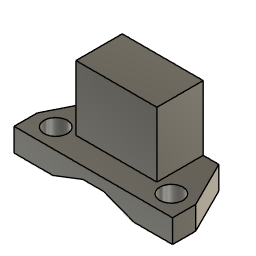
splayFlexJoint (Autodesk Fusion 360 archive; units mm, degrees)
design "hallEffectHolder"
Autodesk Fusion 360 part; units mm, degrees
note: some values were not read from the file. Chosen so that the rebuilt part matches the saved one: that a step has no effect; which face or edge a step refers to. Set by a fixed rule: which sketch regions a step uses.
sketch "mainBase" plane through (0, 0, 0) normal (0, 0, 1) x (1, 0, 0)
  line L0 (0, 0) -> (13.7, 0)
  line L1 (13.7, 0) -> (13.7, 6)
  line L2 (13.7, 6) -> (0, 6)
  line L3 (0, 6) -> (0, 0)
  line L4 (0, 0) -> (6.85, 0)
  line L5 (6.85, 0) -> (6.85, 1.75)
  line L6 (6.85, 1.75) -> (1.85, 1.75)
  line L7 (6.85, 1.75) -> (11.85, 1.75)
  line L8 (0, 6) -> (6.85, 6)
  circle A0 centre (1.85, 1.75) radius 1
  circle A1 centre (11.85, 1.75) radius 1
  line L9 (6.85, 6) -> (3.35, 6)
  line L10 (3.35, 6) -> (3.35, 2)
  line L11 (3.35, 2) -> (6.85, 2)
  line L12 (6.85, 2) -> (6.85, 6)
  line L13 (6.85, 6) -> (10.35, 6)
  line L14 (10.35, 6) -> (10.35, 2)
  line L15 (10.35, 2) -> (6.85, 2)
  line L16 (6.85, 2) -> (6.85, 6)
  dimension "d9" = 6
  dimension "d10" = 13.7
  dimension "d11" = 6.85
  dimension "d12" = 1.75
  dimension "d13" = 5
  dimension "d14" = 5
  dimension "d15" = 6.85
  dimension "d17" = 2
  dimension "d18" = 2
  dimension "d19" = 4
  dimension "d20" = 3.5
  dimension "d21" = 4
  dimension "d22" = 3.5
  constraint horizontal L0
  constraint vertical L1
  constraint horizontal L2
  constraint vertical L3
  constraint coincident L0.start L3.end
  constraint perpendicular L3 L4
  constraint perpendicular L0 L5
  constraint perpendicular L5 L6
  constraint perpendicular L5 L7
  constraint perpendicular L3 L8
  constraint coincident L6.end A0.centre
  constraint coincident L7.end A1.centre
  constraint horizontal L9
  constraint vertical L10
  constraint horizontal L11
  constraint vertical L12
  constraint horizontal L13
  constraint vertical L14
  constraint horizontal L15
  constraint vertical L16
  measures "d9" distance of L0.start L2.end
  measures "d10" distance of L0.start L0.end
  measures "d11" distance of L0.start L4.end
  measures "d12" distance of L4.end L5.end
  measures "d13" distance of L5.end L6.end
  measures "d14" distance of L5.end L7.end
  measures "d15" distance of L2.end L8.end
  measures "d17" diameter of A0
  measures "d18" diameter of A1
  measures "d19" distance of L8.end L11.end
  measures "d20" distance of L10.end L11.end
  measures "d21" distance of L8.end L11.end
  measures "d22" distance of L14.end L11.end
extrude "Extrude1" add sketch "mainBase" along normal blind 7.6 contours L2 L8 L9 L10 L11 L12 L16 | L2 L12 L13 L14 L15 L16
shell "Shell1" thickness 1 removed faces 1 at (8.0167, 4.6667, 0)
extrude "Extrude2" add sketch "mainBase" along normal blind 2 contours L0 L1 L2 L3 L4 L8 L10 L11 L14 L15
sketch "hallCutOut" plane through (0, 0, 0) normal (0, 0, 1) x (1, 0, 0)
  line L0 (0, 6) -> (6.85, 6)
  line L1 (6.85, 6) -> (6.85, 2)
  line L2 (6.85, 2) -> (3.35, 2)
  line L3 (3.35, 2) -> (3.35, 4)
  line L4 (6.85, 2) -> (6.85, 3)
  line L5 (6.85, 3) -> (5.95, 3)
  line L6 (5.95, 3) -> (3.35, 4)
  line L7 (6.85, 3) -> (7.75, 3)
  line L8 (6.85, 2) -> (10.35, 2)
  line L9 (10.35, 2) -> (10.35, 4)
  line L10 (10.35, 4) -> (7.75, 3)
  line L11 (7.75, 3) -> (9.35, 3)
  line L12 (9.35, 3) -> (9.35, 3.6154)
  line L13 (5.95, 3) -> (4.35, 3)
  line L14 (4.35, 3) -> (4.35, 3.6154)
  dimension "d31" = 6.85
  dimension "d32" = 4
  dimension "d33" = 3.5
  dimension "d34" = 2
  dimension "d35" = 1
  dimension "d36" = 0.9
  dimension "d37" = 0.9
  dimension "d38" = 3.5
  dimension "d39" = 2
  constraint horizontal L0
  constraint perpendicular L0 L1
  constraint perpendicular L1 L2
  constraint perpendicular L2 L3
  constraint perpendicular L2 L4
  constraint perpendicular L1 L5
  constraint perpendicular L1 L7
  constraint perpendicular L4 L8
  constraint perpendicular L8 L9
  constraint parallel L7 L11
  constraint coincident L10 L12.end
  constraint perpendicular L11 L12
  constraint perpendicular L1 L13
  constraint coincident L6 L14.end
  constraint perpendicular L13 L14
  measures "d31" distance of L0.start L0.end
  measures "d32" distance of L0.end L1.end
  measures "d33" distance of L1.end L2.end
  measures "d34" distance of L2.end L3.end
  measures "d35" distance of L1.end L4.end
  measures "d36" distance of L4.end L5.end
  measures "d37" distance of L4.end L7.end
  measures "d38" distance of L1.end L8.end
  measures "d39" distance of L8.end L9.end
extrude "Extrude3" add sketch "hallCutOut" along normal blind 6.6 contours L6 L13 L14 | L10 L11 L12
sketch "wireCutOut" plane through (0, 0, 0) normal (0, -1, 0) x (1, 0, 0)
  line L0 (0, 0) -> (13.7, 0)
  line L1 (13.7, 0) -> (13.7, 2)
  line L2 (13.7, 2) -> (0, 2)
  line L3 (0, 2) -> (0, 0)
  line L4 (0, 0) -> (6.85, 0)
  line L5 (6.85, 0) -> (6.85, 1)
  line L6 (6.85, 1) -> (5.95, 1)
  line L7 (6.85, 1) -> (7.75, 1)
  line L8 (6.85, 0) -> (13.7, 0)
  line L9 (6.85, 0) -> (10.35, 0)
  line L10 (6.85, 0) -> (3.35, 0)
  line L11 (7.75, 1) -> (10.35, 0)
  line L12 (5.95, 1) -> (3.35, 0)
  dimension "d42" = 6.85
  dimension "d43" = 1
  dimension "d44" = 0.9
  dimension "d45" = 0.9
  dimension "d46" = 6.85
  dimension "d47" = 3.5
  dimension "d48" = 3.5
  constraint coincident L0.start L3.end
  constraint perpendicular L3 L4
  constraint perpendicular L4 L5
  constraint perpendicular L5 L6
  constraint perpendicular L5 L7
  constraint perpendicular L5 L8
  constraint perpendicular L5 L9
  constraint perpendicular L5 L10
  measures "d42" distance of L0.start L4.end
  measures "d43" distance of L4.end L5.end
  measures "d44" distance of L5.end L6.end
  measures "d45" distance of L5.end L7.end
  measures "d46" distance of L4.end L0.end
  measures "d47" distance of L4.end L9.end
  measures "d48" distance of L4.end L10.end
extrude "Extrude4" cut sketch "wireCutOut" against normal blind 5 contours L0 L4 L5 L6 L10 L12 | L0 L5 L7 L8 L9 L11
sketch "cutOut" plane through (0, 0, 0) normal (0, 0, 1) x (1, 0, 0)
  line L0 (0, 0) -> (13.7, 0)
  line L1 (13.7, 0) -> (13.7, 6)
  line L2 (13.7, 6) -> (0, 6)
  line L3 (0, 6) -> (0, 0)
  line L4 (13.7, 0) -> (13.7, 2)
  line L5 (0, 0) -> (0, 2)
  line L6 (0, 6) -> (2, 6)
  line L7 (13.7, 6) -> (11.7, 6)
  line L8 (0, 2) -> (2, 6)
  line L9 (13.7, 2) -> (11.7, 6)
  dimension "d51" = 6
  dimension "d52" = 13.7
  dimension "d53" = 2
  dimension "d54" = 2
  dimension "d55" = 2
  dimension "d56" = 2
  constraint horizontal L0
  constraint vertical L1
  constraint horizontal L2
  constraint vertical L3
  constraint coincident L0.start L3.end
  constraint perpendicular L0 L4
  constraint perpendicular L0 L5
  constraint coincident L2 L6.end
  constraint perpendicular L1 L7
  measures "d51" distance of L0.start L2.end
  measures "d52" distance of L0.start L0.end
  measures "d53" distance of L0.end L4.end
  measures "d54" distance of L0.start L5.end
  measures "d55" distance of L1.end L7.end
  measures "d56" distance of L2.end L6.end
extrude "Extrude5" cut sketch "cutOut" along normal blind 2 contours L2 L3 L6 L8 | L1 L2 L7 L9
equation "baseLength = 6 mm"
equation "baseWidth = 13.7 mm"
equation "mountingCircleToMountingCircle = 10 mm"
equation "mountingHoleFromEdge = 1.75 mm"
equation "hallEffectWidth = 7 mm"
equation "hallEffectLength = 4 mm"
equation "hallEffectHeight = 7.6 mm"
equation "baseHeight = 2 mm"
equation "d9 = baseLength"
equation "d10 = baseWidth"
equation "d11 = baseWidth / 2"
equation "d12 = mountingHoleFromEdge"
equation "d13 = mountingCircleToMountingCircle / 2"
equation "d14 = mountingCircleToMountingCircle / 2"
equation "d15 = baseWidth / 2"
equation "screwHole = 2 mm"
equation "d17 = screwHole"
equation "d18 = screwHole"
equation "d19 = hallEffectLength"
equation "d20 = hallEffectWidth / 2"
equation "d21 = hallEffectLength"
equation "d22 = hallEffectWidth / 2"
equation "d23 = hallEffectHeight"
equation "hallEffectThickness = 1 mm"
equation "d26 = hallEffectThickness"
equation "d27 = baseHeight"
equation "traingleHeight = 2 mm"
equation "hallEffectMiddleDist = 1.8 mm"
equation "d31 = baseWidth / 2"
equation "d32 = hallEffectLength"
equation "d33 = hallEffectWidth / 2"
equation "d34 = traingleHeight"
equation "d35 = hallEffectThickness"
equation "d36 = hallEffectMiddleDist / 2"
equation "d37 = hallEffectMiddleDist / 2"
equation "d38 = hallEffectWidth / 2"
equation "d39 = traingleHeight"
equation "d40 = hallEffectHeight - hallEffectThickness"
equation "d42 = baseWidth / 2"
equation "d43 = hallEffectThickness"
equation "d44 = hallEffectMiddleDist / 2"
equation "d45 = hallEffectMiddleDist / 2"
equation "d46 = baseWidth / 2"
equation "d47 = hallEffectWidth / 2"
equation "d48 = hallEffectWidth / 2"
equation "d49 = -( baseLength - hallEffectThickness )"
equation "d51 = baseLength"
equation "d52 = baseWidth"
equation "d53 = baseLength / 3"
equation "d54 = baseLength / 3"
equation "d57 = baseHeight"

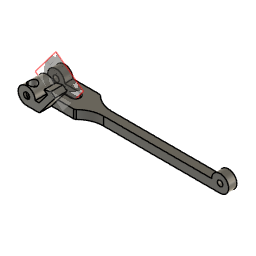
design "bar2Magnet"
Autodesk Fusion 360 part; units mm, degrees
sketch "mainBody" plane through (0, 0, 0) normal (0, 0, 1) x (1, 0, 0)
  line L0 (0, 0) -> (50, 0)
  line L1 (50, 0) -> (50, -1.5)
  line L2 (50, -1.5) -> (0, -1.5)
  line L3 (0, -1.5) -> (0, 0)
  line L4 (0, 0) -> (50, 0)
  line L5 (50, 0) -> (50, 1.5)
  line L6 (50, 1.5) -> (0, 1.5)
  line L7 (0, 1.5) -> (0, 0)
  line L8 (0, 0) -> (-4.4, 0)
  line L9 (-4.4, 0) -> (-4.4, 4.7)
  line L10 (-4.4, 4.7) -> (0, 4.7)
  line L11 (0, 4.7) -> (0, 0)
  line L12 (0, 0) -> (-4.4, 0)
  line L13 (-4.4, 0) -> (-4.4, -4.7)
  line L14 (-4.4, -4.7) -> (0, -4.7)
  line L15 (0, -4.7) -> (0, 0)
  line L16 (-4.4, -4.7) -> (-13.2, -4.7)
  line L17 (-13.2, -4.7) -> (-13.2, -1.7)
  line L18 (-13.2, -1.7) -> (-4.4, -1.7)
  line L19 (-4.4, -1.7) -> (-4.4, -4.7)
  line L20 (-4.4, 4.7) -> (-13.2, 4.7)
  line L21 (-13.2, 4.7) -> (-13.2, 1.7)
  line L22 (-13.2, 1.7) -> (-4.4, 1.7)
  line L23 (-4.4, 1.7) -> (-4.4, 4.7)
  line L24 (50, -1.5) -> (46.25, -1.5)
  line L25 (46.25, -1.5) -> (39.25, -1.5)
  line L26 (39.25, -1.5) -> (39.25, -0.5)
  line L27 (39.25, -0.5) -> (46.25, -0.5)
  line L28 (46.25, -0.5) -> (46.25, -1.5)
  dimension "d10" = 1.5
  dimension "d11" = 50
  dimension "d12" = 50
  dimension "d13" = 1.5
  dimension "d14" = 4.7
  dimension "d15" = 4.7
  dimension "d16" = 4.4
  dimension "d17" = 4.4
  dimension "d18" = 3
  dimension "d19" = 8.8
  dimension "d20" = 8.8
  dimension "d21" = 3
  dimension "d25" = 3.75
  dimension "d26" = 1
  dimension "d27" = 7
  dimension "d68" = 3.4
  constraint horizontal L0
  constraint vertical L1
  constraint horizontal L2
  constraint vertical L3
  constraint coincident L0.start L3.end
  constraint horizontal L4
  constraint vertical L5
  constraint horizontal L6
  constraint vertical L7
  constraint horizontal L8
  constraint vertical L9
  constraint horizontal L10
  constraint vertical L11
  constraint horizontal L12
  constraint vertical L13
  constraint horizontal L14
  constraint vertical L15
  constraint horizontal L16
  constraint vertical L17
  constraint horizontal L18
  constraint vertical L19
  constraint horizontal L20
  constraint vertical L21
  constraint horizontal L22
  constraint vertical L23
  constraint perpendicular L1 L24
  constraint horizontal L25
  constraint vertical L26
  constraint horizontal L27
  constraint vertical L28
  measures "d10" distance of L0.start L2.end
  measures "d11" distance of L1.end L2.end
  measures "d12" distance of L5.end L6.end
  measures "d13" distance of L0.start L6.end
  measures "d14" distance of L0.start L10.end
  measures "d15" distance of L0.start L14.end
  measures "d16" distance of L9.end L10.end
  measures "d17" distance of L13.end L14.end
  measures "d18" distance of L13.end L18.end
  measures "d19" distance of L13.end L16.end
  measures "d20" distance of L9.end L20.end
  measures "d21" distance of L20.end L21.end
  measures "d25" distance of L1.end L24.end
  measures "d26" distance of L24.end L27.end
  measures "d27" distance of L24.end L25.end
  measures "d68" distance of L18.end L22.end
extrude "Extrude1" add sketch "mainBody" along normal blind 3.125 contours L0 L4 L5 L6 L7 L11 | L0 L1 L2 L3 L4 L15 L24 L26 L27 L28 | L7 L8 L9 L10 L11 L12 L23 | L3 L8 L12 L13 L14 L15 L19 | L9 L20 L21 L22 L23 | L13 L16 L17 L18 L19
sketch "backHole" plane through (0, -1.5, 0) normal (0, -1, 0) x (1, 0, 0)
  line L0 (0, 0) -> (39.25, 0)
  line L1 (39.25, 0) -> (39.25, 3.125)
  line L2 (39.25, 3.125) -> (0, 3.125)
  line L3 (0, 3.125) -> (0, 0)
  circle A0 centre (50, 3.125) radius 3.125
  circle A1 centre (50, 3.125) radius 1
  line L4 (0, 0) -> (50, 0)
  line L5 (50, 0) -> (50, 3.125)
  line L6 (50, 3.125) -> (0, 3.125)
  line L7 (0, 3.125) -> (0, 0)
  dimension "d30" = 6.25
  dimension "d31" = 2
  dimension "d65" = 50
  dimension "d66" = 3.125
  constraint concentric A0 A1
  constraint horizontal L4
  constraint vertical L5
  constraint horizontal L6
  constraint vertical L7
  constraint coincident A0.centre A1.centre
  constraint coincident L0.start L3.end
  measures "d30" diameter of A0
  measures "d31" diameter of A1
  measures "d65" distance of L0.start L4.end
  measures "d66" distance of L0.start L2.end
extrude "Extrude2" cut sketch "backHole" against normal blind 3 contours A1 L5 L6 | A1 L5 L6
extrude "Extrude3" add sketch "backHole" against normal blind 3 contours A0 A1 L5 L6 | A0 A1 L5 L6
sketch "oneFrontHole" plane through (0, -1.7, 0) normal (0, 1, 0) x (-1, 0, 0)
  line L0 (4.4, 0) -> (13.2, 0)
  line L1 (13.2, 0) -> (13.2, 3.125)
  line L2 (13.2, 3.125) -> (4.4, 3.125)
  line L3 (4.4, 3.125) -> (4.4, 0)
  circle A0 centre (13.2, 3.125) radius 3.125
  circle A1 centre (13.2, 3.125) radius 1.1
  line L4 (13.2, 0) -> (0, 0)
  dimension "d40" = 6.25
  dimension "d41" = 2.2
  dimension "d74" = 13.2
  dimension "d75" = 3.125
  constraint coincident L1.end L2.start
  constraint concentric A0 A1
  measures "d40" diameter of A0
  measures "d41" diameter of A1
  measures "d74" distance of L0.end L4.end
  measures "d75" distance of L0.end L1.end
extrude "Extrude4" cut sketch "oneFrontHole" against normal blind 3 contours L1 L2 A1 picked at (12.4704, 3.0728)
extrude "Extrude5" add sketch "oneFrontHole" against normal blind 3 contours L1 L2 A0 A1 picked at (12.4537, 5.4515)
sketch "twoFrontHole" plane through (0, 1.7, 0) normal (0, -1, 0) x (1, 0, 0)
  line L0 (-13.2, 0) -> (-4.4, 0)
  line L1 (-4.4, 0) -> (-4.4, 3.125)
  line L2 (-4.4, 3.125) -> (-13.2, 3.125)
  line L3 (-13.2, 3.125) -> (-13.2, 0)
  circle A0 centre (-13.2, 3.125) radius 3.125
  circle A1 centre (-13.2, 3.125) radius 1.1
  dimension "d46" = 6.25
  dimension "d47" = 2.2
  constraint coincident L2.end L3.start
  measures "d46" diameter of A0
  measures "d47" diameter of A1
extrude "Extrude6" cut sketch "twoFrontHole" against normal blind 3 contours L2 L3 A1 picked at (-12.4704, 3.0728)
extrude "Extrude7" add sketch "twoFrontHole" against normal blind 3 contours L2 L3 A0 A1 picked at (-14.7245, 1.2154)
extrude "Extrude8" add sketch "mainBody" along normal blind 3.125 contours L2 L25 L26 L27 L28
fillet "Fillet1" radius 10 1 edges at (0, -1.5, 1.5625)
fillet "Fillet2" radius 10 1 edges at (0, 1.5, 1.5625)
fillet "Fillet3" radius 1 2 edges at (0, 4.7, 1.5625) (0, -4.7, 1.5625)
fillet "Fillet4" [no effect]
fillet "Fillet5" [no effect]
sketch "roundedInside" plane through (0, 0, 3.125) normal (0, 0, 1) x (-1, 0, 0)
  line L0 (10.075, -4.7) -> (10.075, -1.7)
  line L1 (10.075, -1.7) -> (4.4, -1.7)
  line L2 (4.4, -1.7) -> (4.4, 1.7)
  line L3 (4.4, 1.7) -> (10.075, 1.7)
  line L4 (10.075, 1.7) -> (10.075, 4.7)
  line L5 (-46.875, 1.5) -> (-46.875, -1.5)
  circle A0 centre (4.4, 0) radius 1.7
  arc A1 (0.4242, 4.7) -> (-0.281, 4.4091) centre (0.4242, 3.7) ccw
  arc A2 (-7.3321, 1.5) -> (-0.281, 4.4091) centre (-7.3321, 11.5) ccw
  line L6 (-7.3321, 1.5) -> (-46.875, 1.5)
  line L7 (-46.875, -1.5) -> (-7.3321, -1.5)
  arc A3 (-0.281, -4.4091) -> (-7.3321, -1.5) centre (-7.3321, -11.5) ccw
  arc A4 (-0.281, -4.4091) -> (0.4242, -4.7) centre (0.4242, -3.7) ccw
  line L8 (0.4242, -4.7) -> (10.075, -4.7)
  line L9 (10.075, 4.7) -> (0.4242, 4.7)
  dimension "d69" = 3.4
  constraint midpoint L2 A0.centre
  measures "d69" diameter of A0
extrude "Extrude9" cut sketch "roundedInside" against normal blind 3.125 contours L2 A0 | L2 A0
fillet "Fillet6" [no effect]
sketch "magnet" plane through (0, -4.7, 0) normal (0, -1, 0) x (1, 0, 0)
  line L0 (-0.4242, 0) -> (-0.4242, 3.125)
  line L1 (-0.4242, 3.125) -> (-10.075, 3.125)
  arc A0 (-10.075, 3.125) -> (-13.2, 0) centre (-13.2, 3.125) ccw
  line L2 (-13.2, 0) -> (-0.4242, 0)
  circle A1 centre (-13.2, 3.125) radius 1.1
  line L3 (0, 0) -> (-13.2, 0)
  line L4 (-13.2, 0) -> (-13.2, 3.125)
  line L5 (-13.2, 3.125) -> (0, 3.125)
  line L6 (0, 3.125) -> (0, 0)
  circle A2 centre (-13.2, 3.125) radius 3.125
  dimension "d76" = 6.25
  constraint horizontal L3
  constraint vertical L4
  constraint horizontal L5
  constraint vertical L6
  constraint coincident A0.centre A1.centre
  constraint coincident L3.start L6.end
  constraint concentric A0 A2
  measures "d76" diameter of A2
extrude "Extrude10" add sketch "magnet" along normal blind 4.4 contours A0 A1 L4 L5 A2 | A1 L4 L5 A2 | A1 L4 L5 | A1 L4 L5
hole "Hole1" at (-15.4097, -6.754, 5.3347) direction (0.707107, 0, -0.707107) diameter 1 depth 4 tip angle 180
extrude "Extrude11" add 1 faces at (-12.374, -9.1, 3.2495) along direction (0, 1, 0) blind 4.4
hole "Hole2" at (-10.9903, -6.7983, 5.3347) direction (-0.707107, 0, -0.707107) diameter 3.2 depth 7.8 tip angle 180
sketch "Sketch9" plane through (0, -4.7, 0) normal (0, -1, 0) x (1, 0, 0)
  arc A0 (-13.2, 0) -> (-10.075, 3.125) centre (-13.2, 3.125) ccw
  line L0 (-13.2, 0) -> (-0.4242, 0)
  line L1 (-0.4242, 0) -> (-0.4242, 3.125)
  line L2 (-0.4242, 3.125) -> (-10.075, 3.125)
  line L3 (-10.075, 3.125) -> (-13, 0)
  line L4 (-13, 0) -> (-11, 0)
  line L5 (-10.075, 3.125) -> (-8.075, 3.125)
  line L6 (-11, 0) -> (-8.075, 3.125)
  line L7 (-10.075, 3.125) -> (-4.4181, 8.7819)
  line L8 (-8.075, 3.125) -> (-2.6081, 8.9657)
  line L9 (-4.4181, 8.7819) -> (-2.6081, 8.9657)
  line L10 (-4.4181, 8.7819) -> (-5.8324, 10.1961)
  line L11 (-2.6081, 8.9657) -> (-5.8324, 10.1961)
  dimension "d92" = 2
  dimension "d93" = 2
  dimension "d95" = 8
  dimension "d96" = 8
  dimension "d98" = 2
  constraint coincident A0.end L2.end
  constraint coincident L0 L3.end
  constraint parallel L0 L4
  constraint parallel L2 L5
  constraint parallel L6 L8
  constraint perpendicular L7 L10
  measures "d92" distance of L3.end L4.end
  measures "d93" distance of A0.end L5.end
  measures "d95" distance of A0.end L7.end
  measures "d96" distance of L5.end L8.end
  measures "d98" distance of L7.end L10.end
extrude "Extrude12" add sketch "Sketch9" along normal blind 4.4 contours A0 L0 L2 L3 L4 L5 L6 | L2 L5 L7 L8 L9 | L9 L10 L11
extrude "Extrude13" add sketch "magnet" along normal blind 4.4 contours A0 A1 L4 L5 A2 | A1 L4 L5 A2 | A1 L4 L5 | A1 L4 L5
hole "Hole3" at (-13.2, -7.0048, 0) direction (0, 0, 1) diameter 3.2 depth 6.25 tip angle 180
extrude "Extrude14" cut 1 faces at (-13.5393, -4.7, 3.4906) along direction (0, -1, 0) blind 4.4
extrude "Extrude15" cut sketch "Sketch9" along normal blind 4.4 contours A0 L0 L2 L3 L4 L5 L6 | L2 L5 L7 L8 L9 | L9 L10 L11
sketch "Sketch12" plane through (0, -4.7, 0) normal (0, -1, 0) x (1, 0, 0)
  line L0 (-13.2, 0) -> (-0.4242, 0)
  line L1 (-0.4242, 0) -> (-0.4242, 3.125)
  line L2 (-0.4242, 3.125) -> (-10.075, 3.125)
  arc A0 (-13.2, 0) -> (-10.075, 3.125) centre (-13.2, 3.125) ccw
  line L3 (-5.675, 7.2) -> (-8.0564, 4.0395)
  line L4 (-8.0564, 4.0395) -> (-13.6194, 8.2311)
  line L5 (-13.6194, 8.2311) -> (-11.2359, 11.3943)
  line L6 (-11.2359, 11.3943) -> (-5.675, 7.2)
  line L7 (-5.675, 7.2) -> (-5.575, 7.2)
  line L8 (-5.575, 7.2) -> (-8, 4)
  line L9 (-8, 4) -> (-11.0312, 0)
  line L10 (-11.2359, 11.3943) -> (-11.2359, 11.4943)
  line L11 (-5.575, 7.2) -> (-4.3663, 8.7934)
  line L12 (-5.575, 7.2) -> (-3.9816, 5.9913)
  line L13 (-3.9816, 5.9913) -> (-2.7729, 7.5847)
  line L14 (-3.9816, 5.9913) -> (-8.5265, 0)
  line L15 (-8.5265, 0) -> (-11.0312, 0)
  line L16 (-5.575, 7.2) -> (-6.8689, 8.1816)
  line L17 (-6.8689, 8.1816) -> (-4.3663, 8.7934)
  line L18 (-4.3663, 8.7934) -> (-2.7729, 7.5847)
  dimension "d111" = 0.1
  dimension "d112" = 0.1
  dimension "d115" = 2
  dimension "d116" = 2
  dimension "d117" = 2
  constraint perpendicular L3 L4
  constraint perpendicular L4 L5
  constraint horizontal L7
  constraint coincident L0 L9.end
  constraint parallel L8 L9
  constraint vertical L10
  constraint perpendicular L11 L12
  constraint perpendicular L12 L13
  constraint coincident L0 L14.end
  constraint perpendicular L12 L14
  constraint perpendicular L11 L16
  measures "d111" distance of L3.start L7.end
  measures "d112" distance of L5.end L10.end
  measures "d115" distance of L7.end L11.end
  measures "d116" distance of L7.end L12.end
  measures "d117" distance of L12.end L13.end
extrude "Extrude16" add sketch "Sketch12" along normal blind 4.4 contours L0 L2 A0 L9 | L0 L2 L9 L14 L15 | L2 L8 L9 L12 L14 | L11 L12 L13 L18 | L11 L16 L17
hole "Hole4" at (-13.2, -7.0134, 6.25) direction (0, 0, -1) diameter 3.2 depth 7 tip angle 118
equation "mainBarLength = 50 mm" comment "50mm"
equation "mainBarWidth = 3 mm"
equation "mainBarHeight = 3.125 mm"
equation "tBarLength = 9.4 mm"
equation "tBarWidth = 4.4 mm"
equation "hBarHeight = 8.8 mm" comment "6.8mm"
equation "hBarWidth = 3 mm"
equation "outerCircle = 6.25 mm"
equation "innerCircle = 2.2 mm"
equation "d10 = mainBarWidth / 2"
equation "d11 = mainBarLength"
equation "d12 = mainBarLength"
equation "d13 = mainBarWidth / 2"
equation "d14 = tBarLength / 2"
equation "d15 = tBarLength / 2"
equation "d16 = tBarWidth"
equation "d17 = tBarWidth"
equation "d18 = hBarWidth"
equation "d19 = hBarHeight"
equation "d20 = hBarHeight"
equation "d21 = hBarWidth"
equation "insertDist = 3.75 mm"
equation "insertWidth = 7 mm"
equation "insertHeight = 1 mm"
equation "d25 = insertDist"
equation "d26 = insertHeight"
equation "d27 = insertWidth"
equation "d28 = mainBarHeight"
equation "d30 = outerCircle"
equation "d31 = innerCircleSmallDiam"
equation "d34 = -mainBarWidth"
equation "d36 = -mainBarWidth"
equation "d40 = outerCircle"
equation "d41 = innerCircle"
equation "d42 = -hBarWidth"
equation "d44 = -hBarWidth"
equation "d46 = outerCircle"
equation "d47 = innerCircle"
equation "d48 = -hBarWidth"
equation "d50 = -hBarWidth"
equation "d52 = mainBarHeight"
equation "pointerFingerOffset = 25 mm"
equation "d65 = mainBarLength"
equation "d66 = mainBarHeight"
equation "innerCircleSmallDiam = 2 mm"
equation "d70 = -mainBarHeight"
equation "d76 = outerCircle"
equation "magnetAddittionDepth = 4.4 mm"
equation "magnetDiam = 3.2 mm"
equation "magnetDepth = 4 mm"
equation "d80 = magnetAddittionDepth"
equation "d82 = magnetDepth"
equation "d85 = -magnetAddittionDepth"
equation "d88 = magnetDiam"
equation "holedegrees = 180 deg"
equation "caseThickness = 2 mm"
equation "d92 = caseThickness"
equation "d93 = caseThickness"
equation "hookLength = 8 mm"
equation "d95 = hookLength"
equation "d96 = hookLength"
equation "clipHang = 2 mm"
equation "d98 = clipHang"
equation "d99 = magnetAddittionDepth"
equation "d101 = magnetAddittionDepth"
equation "d103 = outerCircle"
equation "d104 = magnetDiam"
equation "d106 = -magnetAddittionDepth"
equation "d108 = magnetAddittionDepth"
equation "tolerance = 0.1 mm"
equation "d111 = tolerance"
equation "d112 = tolerance"
equation "d115 = caseThickness"
equation "d116 = caseThickness"
equation "d117 = caseThickness"
equation "d118 = magnetAddittionDepth"
equation "d121 = magnetDiam"

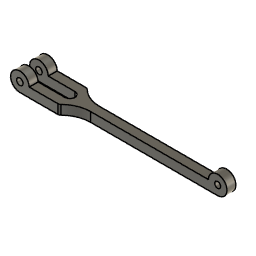
design "bar2"
Autodesk Fusion 360 part; units mm, degrees
sketch "mainBody" plane through (0, 0, 0) normal (0, 0, 1) x (1, 0, 0)
  line L0 (0, 0) -> (50, 0)
  line L1 (50, 0) -> (50, -1.5)
  line L2 (50, -1.5) -> (0, -1.5)
  line L3 (0, -1.5) -> (0, 0)
  line L4 (0, 0) -> (50, 0)
  line L5 (50, 0) -> (50, 1.5)
  line L6 (50, 1.5) -> (0, 1.5)
  line L7 (0, 1.5) -> (0, 0)
  line L8 (0, 0) -> (-1.1, 0)
  line L9 (-1.1, 0) -> (-1.1, 4.7)
  line L10 (-1.1, 4.7) -> (0, 4.7)
  line L11 (0, 4.7) -> (0, 0)
  line L12 (0, 0) -> (-1.1, 0)
  line L13 (-1.1, 0) -> (-1.1, -4.7)
  line L14 (-1.1, -4.7) -> (0, -4.7)
  line L15 (0, -4.7) -> (0, 0)
  line L16 (-1.1, -4.7) -> (-13.2, -4.7)
  line L17 (-13.2, -4.7) -> (-13.2, -1.7)
  line L18 (-13.2, -1.7) -> (-1.1, -1.7)
  line L19 (-1.1, -1.7) -> (-1.1, -4.7)
  line L20 (-1.1, 4.7) -> (-13.2, 4.7)
  line L21 (-13.2, 4.7) -> (-13.2, 1.7)
  line L22 (-13.2, 1.7) -> (-1.1, 1.7)
  line L23 (-1.1, 1.7) -> (-1.1, 4.7)
  line L24 (50, -1.5) -> (46.25, -1.5)
  line L25 (46.25, -1.5) -> (39.25, -1.5)
  line L26 (39.25, -1.5) -> (39.25, -0.5)
  line L27 (39.25, -0.5) -> (46.25, -0.5)
  line L28 (46.25, -0.5) -> (46.25, -1.5)
  dimension "d10" = 1.5
  dimension "d11" = 50
  dimension "d12" = 50
  dimension "d13" = 1.5
  dimension "d14" = 4.7
  dimension "d15" = 4.7
  dimension "d16" = 1.1
  dimension "d17" = 1.1
  dimension "d18" = 3
  dimension "d19" = 12.1
  dimension "d20" = 12.1
  dimension "d21" = 3
  dimension "d25" = 3.75
  dimension "d26" = 1
  dimension "d27" = 7
  dimension "d68" = 3.4
  constraint horizontal L0
  constraint vertical L1
  constraint horizontal L2
  constraint vertical L3
  constraint coincident L0.start L3.end
  constraint horizontal L4
  constraint vertical L5
  constraint horizontal L6
  constraint vertical L7
  constraint horizontal L8
  constraint vertical L9
  constraint horizontal L10
  constraint vertical L11
  constraint horizontal L12
  constraint vertical L13
  constraint horizontal L14
  constraint vertical L15
  constraint horizontal L16
  constraint vertical L17
  constraint horizontal L18
  constraint vertical L19
  constraint horizontal L20
  constraint vertical L21
  constraint horizontal L22
  constraint vertical L23
  constraint perpendicular L1 L24
  constraint horizontal L25
  constraint vertical L26
  constraint horizontal L27
  constraint vertical L28
  measures "d10" distance of L0.start L2.end
  measures "d11" distance of L1.end L2.end
  measures "d12" distance of L5.end L6.end
  measures "d13" distance of L0.start L6.end
  measures "d14" distance of L0.start L10.end
  measures "d15" distance of L0.start L14.end
  measures "d16" distance of L9.end L10.end
  measures "d17" distance of L13.end L14.end
  measures "d18" distance of L13.end L18.end
  measures "d19" distance of L13.end L16.end
  measures "d20" distance of L9.end L20.end
  measures "d21" distance of L20.end L21.end
  measures "d25" distance of L1.end L24.end
  measures "d26" distance of L24.end L27.end
  measures "d27" distance of L24.end L25.end
  measures "d68" distance of L18.end L22.end
extrude "Extrude1" add sketch "mainBody" along normal blind 3.125 contours L0 L4 L5 L6 L7 L11 | L0 L1 L2 L3 L4 L15 L24 L26 L27 L28 | L7 L8 L9 L10 L11 L12 L23 | L3 L8 L12 L13 L14 L15 L19 | L9 L20 L21 L22 L23 | L13 L16 L17 L18 L19
sketch "backHole" plane through (0, -1.5, 0) normal (0, -1, 0) x (1, 0, 0)
  line L0 (0, 0) -> (39.25, 0)
  line L1 (39.25, 0) -> (39.25, 3.125)
  line L2 (39.25, 3.125) -> (0, 3.125)
  line L3 (0, 3.125) -> (0, 0)
  circle A0 centre (50, 3.125) radius 3.125
  circle A1 centre (50, 3.125) radius 1
  line L4 (0, 0) -> (50, 0)
  line L5 (50, 0) -> (50, 3.125)
  line L6 (50, 3.125) -> (0, 3.125)
  line L7 (0, 3.125) -> (0, 0)
  dimension "d30" = 6.25
  dimension "d31" = 2
  dimension "d65" = 50
  dimension "d66" = 3.125
  constraint concentric A0 A1
  constraint horizontal L4
  constraint vertical L5
  constraint horizontal L6
  constraint vertical L7
  constraint coincident A0.centre A1.centre
  constraint coincident L0.start L3.end
  measures "d30" diameter of A0
  measures "d31" diameter of A1
  measures "d65" distance of L0.start L4.end
  measures "d66" distance of L0.start L2.end
extrude "Extrude2" cut sketch "backHole" against normal blind 3 contours A1 L5 L6 | A1 L5 L6
extrude "Extrude3" add sketch "backHole" against normal blind 3 contours A0 A1 L5 L6 | A0 A1 L5 L6
sketch "oneFrontHole" plane through (0, -1.7, 0) normal (0, 1, 0) x (-1, 0, 0)
  line L0 (1.1, 0) -> (13.2, 0)
  line L1 (13.2, 0) -> (13.2, 3.125)
  line L2 (13.2, 3.125) -> (1.1, 3.125)
  line L3 (1.1, 3.125) -> (1.1, 0)
  circle A0 centre (13.2, 3.125) radius 3.125
  circle A1 centre (13.2, 3.125) radius 1.1
  dimension "d40" = 6.25
  dimension "d41" = 2.2
  constraint coincident L1.end L2.start
  constraint concentric A0 A1
  measures "d40" diameter of A0
  measures "d41" diameter of A1
extrude "Extrude4" cut sketch "oneFrontHole" against normal blind 3 contours L1 L2 A1 picked at (12.4704, 3.0728)
extrude "Extrude5" add sketch "oneFrontHole" against normal blind 3 contours L1 L2 A0 A1 picked at (12.4537, 5.4515)
sketch "twoFrontHole" plane through (0, 1.7, 0) normal (0, -1, 0) x (1, 0, 0)
  line L0 (-13.2, 0) -> (-1.1, 0)
  line L1 (-1.1, 0) -> (-1.1, 3.125)
  line L2 (-1.1, 3.125) -> (-13.2, 3.125)
  line L3 (-13.2, 3.125) -> (-13.2, 0)
  circle A0 centre (-13.2, 3.125) radius 3.125
  circle A1 centre (-13.2, 3.125) radius 1.1
  dimension "d46" = 6.25
  dimension "d47" = 2.2
  constraint coincident L2.end L3.start
  measures "d46" diameter of A0
  measures "d47" diameter of A1
extrude "Extrude6" cut sketch "twoFrontHole" against normal blind 3 contours L2 L3 A1 picked at (-12.4704, 3.0728)
extrude "Extrude7" add sketch "twoFrontHole" against normal blind 3 contours L2 L3 A0 A1 picked at (-14.7245, 1.2154)
extrude "Extrude8" add sketch "mainBody" along normal blind 3.125 contours L2 L25 L26 L27 L28
fillet "Fillet1" radius 10 1 edges at (0, -1.5, 1.5625)
fillet "Fillet2" radius 10 1 edges at (0, 1.5, 1.5625)
fillet "Fillet3" radius 1 2 edges at (0, 4.7, 1.5625) (0, -4.7, 1.5625)
fillet "Fillet4" [no effect]
fillet "Fillet5" [no effect]
sketch "Sketch7" plane through (0, 0, 3.125) normal (0, 0, 1) x (-1, 0, 0)
  line L0 (10.075, -4.7) -> (10.075, -1.7)
  line L1 (10.075, -1.7) -> (1.1, -1.7)
  line L2 (1.1, -1.7) -> (1.1, 1.7)
  line L3 (1.1, 1.7) -> (10.075, 1.7)
  line L4 (10.075, 1.7) -> (10.075, 4.7)
  line L5 (-46.875, 1.5) -> (-46.875, -1.5)
  circle A0 centre (1.1, 0) radius 1.7
  arc A1 (0.4242, 4.7) -> (-0.281, 4.4091) centre (0.4242, 3.7) ccw
  arc A2 (-7.3321, 1.5) -> (-0.281, 4.4091) centre (-7.3321, 11.5) ccw
  line L6 (-7.3321, 1.5) -> (-46.875, 1.5)
  line L7 (-46.875, -1.5) -> (-7.3321, -1.5)
  arc A3 (-0.281, -4.4091) -> (-7.3321, -1.5) centre (-7.3321, -11.5) ccw
  arc A4 (-0.281, -4.4091) -> (0.4242, -4.7) centre (0.4242, -3.7) ccw
  line L8 (0.4242, -4.7) -> (10.075, -4.7)
  line L9 (10.075, 4.7) -> (0.4242, 4.7)
  dimension "d69" = 3.4
  constraint midpoint L2 A0.centre
  measures "d69" diameter of A0
extrude "Extrude9" cut sketch "Sketch7" against normal blind 3.125 contours L2 A0 | L2 A0
fillet "Fillet6" [no effect]
equation "mainBarLength = 50 mm"
equation "mainBarWidth = 3 mm"
equation "mainBarHeight = 3.125 mm"
equation "tBarLength = 9.4 mm"
equation "tBarWidth = 4.4 mm"
equation "hBarHeight = 8.8 mm" comment "6.8mm"
equation "hBarWidth = 3 mm"
equation "outerCircle = 6.25 mm"
equation "innerCircle = 2.2 mm"
equation "d10 = mainBarWidth / 2"
equation "d11 = mainBarLength"
equation "d12 = mainBarLength"
equation "d13 = mainBarWidth / 2"
equation "d14 = tBarLength / 2"
equation "d15 = tBarLength / 2"
equation "d16 = tBarWidth / 4"
equation "d17 = tBarWidth / 4"
equation "d18 = hBarWidth"
equation "d19 = hBarHeight + tBarWidth * 3 / 4"
equation "d20 = hBarHeight + tBarWidth * 3 / 4"
equation "d21 = hBarWidth"
equation "insertDist = 3.75 mm"
equation "insertWidth = 7 mm"
equation "insertHeight = 1 mm"
equation "d25 = insertDist"
equation "d26 = insertHeight"
equation "d27 = insertWidth"
equation "d28 = mainBarHeight"
equation "d30 = outerCircle"
equation "d31 = innerCircleSmallDiam"
equation "d34 = -mainBarWidth"
equation "d36 = -mainBarWidth"
equation "d40 = outerCircle"
equation "d41 = innerCircle"
equation "d42 = -hBarWidth"
equation "d44 = -hBarWidth"
equation "d46 = outerCircle"
equation "d47 = innerCircle"
equation "d48 = -hBarWidth"
equation "d50 = -hBarWidth"
equation "d52 = mainBarHeight"
equation "pointerFingerOffset = 25 mm"
equation "d65 = mainBarLength"
equation "d66 = mainBarHeight"
equation "innerCircleSmallDiam = 2 mm"
equation "d70 = -mainBarHeight"
